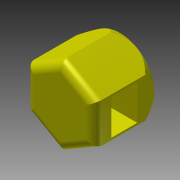
# Autodesk Inventor part: bottom nut
Saved by Autodesk Inventor 2013 (Build 170138000, 138)
## iProperties
Created: 2013-12-06
Part Number: bottom nut
Material: Generic
Document SubType Name: Modeling
Designer: employee
Density: 1 g/cm^3
Author: employee
Autodesk Inventor part; units mm, degrees
ref_plane "YZ Plane" through (0, 0, 0) normal (1, 0, 0) x (0, 1, 0)
ref_plane "XZ Plane" through (0, 0, 0) normal (0, 1, 0) x (-1, 0, 0)
ref_plane "XY Plane" through (0, 0, 0) normal (0, 0, 1) x (1, 0, 0)
sketch "Sketch1" plane through (0, 0, 0) normal (0, 0, 1) x (1, 0, 0)
  line L0 (0, 14.6647) -> (12.7, 7.3323)
  line L1 (12.7, 7.3323) -> (12.7, -7.3323)
  line L2 (12.7, -7.3323) -> (0, -14.6647)
  line L3 (0, -14.6647) -> (-12.7, -7.3323)
  line L4 (-12.7, -7.3323) -> (-12.7, 7.3323)
  line L5 (-12.7, 7.3323) -> (0, 14.6647)
  point P0 (0, 0)
  point P1 (0, 0)
  dimension "d0" = 25.4
  constraints: 12 end point, 1 coincident, 1 vertical, 13 other
  measures "d0" distance between parallel lines of L1 L4
extrude "Extrusion1" add sketch "Sketch1" along normal blind 6.35
sketch "Sketch2" plane through (0, 0, 6.35) normal (0, 0, 1) x (1, 0, 0)
  line L0 (12.7, 7.3323) -> (0, 14.6647) projected
  line L1 (0, 14.6647) -> (-12.7, 7.3323) projected
  line L2 (-12.7, 7.3323) -> (-12.7, -7.3323) projected
  line L3 (-12.7, -7.3323) -> (0, -14.6647) projected
  line L4 (0, -14.6647) -> (12.7, -7.3323) projected
  line L5 (12.7, -7.3323) -> (12.7, 7.3323) projected
  line L6 (7.5523, 0) -> (3.7762, -6.5405)
  line L7 (3.7762, -6.5405) -> (-3.7762, -6.5405)
  line L8 (-3.7762, -6.5405) -> (-7.5523, 0)
  line L9 (-7.5523, 0) -> (-3.7762, 6.5405)
  line L10 (-3.7762, 6.5405) -> (3.7762, 6.5405)
  line L11 (3.7762, 6.5405) -> (7.5523, 0)
  line L12 (3.7762, 6.5405) -> (12.7, 6.5405)
  line L13 (3.7762, -6.5405) -> (12.7, -6.5405)
  point P0 (0, 0)
  point P1 (0, 0)
  dimension "d3" = 13.081
  constraints: 16 end point, 2 point on line, 1 coincident, 1 horizontal, 1 parallel, 1 perpendicular, 13 other
  measures "d3" distance between parallel lines of L7 L10
extrude "Extrusion2" add sketch "Sketch2" along normal blind 9.525 contours L5 L12 L10 L9 L8 L7 L13 L4 L3 L2 L1 L0
sketch "Sketch3" plane through (0, 0, 15.875) normal (0, 0, 1) x (1, 0, 0)
  line L0 (12.7, 7.3323) -> (0, 14.6647) projected
  line L1 (0, 14.6647) -> (-12.7, 7.3323) projected
  line L2 (-12.7, 7.3323) -> (-12.7, -7.3323) projected
  line L3 (-12.7, -7.3323) -> (0, -14.6647) projected
  line L4 (0, -14.6647) -> (12.7, -7.3323) projected
  line L5 (12.7, -7.3323) -> (12.7, -6.5405) projected
  line L6 (12.7, -6.5405) -> (-3.7762, -6.5405) projected
  line L7 (-3.7762, -6.5405) -> (-7.5523, 0) projected
  line L8 (-7.5523, 0) -> (-3.7762, 6.5405) projected
  line L9 (-3.7762, 6.5405) -> (12.7, 6.5405) projected
  line L10 (12.7, 6.5405) -> (12.7, 7.3323) projected
  line L11 (12.7, 6.5405) -> (12.7, -6.5405)
  point P0 (0, 0)
  constraints: 2 end point, 1 collinear
extrude "Extrusion3" add sketch "Sketch3" along normal blind 6.35
sketch "Sketch4" plane through (0, 0, 0) normal (0, 0, -1) x (-1, 0, 0)
  circle A0 centre (0, 0) radius 12.7
  line L0 (0, 14.6647) -> (-12.7, 7.3323) projected
  constraints: 1 centre point, 1 coincident, 1 tangent
extrude "Extrusion4" cut sketch "Sketch4" against normal through all draft 30 keep common part
sketch "Sketch5" plane through (0, 0, 0) normal (0, 0, -1) x (-1, 0, 0)
  circle A0 centre (0, 0) radius 12.7
  circle A1 centre (0, 0) radius 4.3656
  arc A2 (-12.7, 0) -> (-6.35, -10.9985) centre (0, 0) ccw projected
  arc A3 (-6.35, -10.9985) -> (6.35, -10.9985) centre (0, 0) ccw projected
  arc A4 (6.35, -10.9985) -> (12.7, 0) centre (0, 0) ccw projected
  arc A5 (12.7, 0) -> (6.35, 10.9985) centre (0, 0) ccw projected
  arc A6 (6.35, 10.9985) -> (-6.35, 10.9985) centre (0, 0) ccw projected
  arc A7 (-6.35, 10.9985) -> (-12.7, 0) centre (0, 0) ccw projected
  dimension "d13" = 8.7312
  constraints: 2 centre point, 1 coincident
  measures "d13" diameter of A1
extrude "Extrusion5" cut sketch "Sketch5" against normal up to next contours A1
fillet "Fillet1" radius 3.175 6 edges at (12.7, 0, 22.225) (6.35, 10.9985, 22.225) (-6.35, 10.9985, 22.225) (-12.7, 0, 22.225) (-6.35, -10.9985, 22.225) (6.35, -10.9985, 22.225)
body "Solid1"
